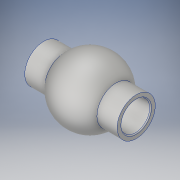
# Autodesk Inventor part: Bola_de_libertad_menor
Saved by Autodesk Inventor 2019 (Build 230136000, 136)
## iProperties
Created: 2019-09-21
Part Number: Bola_de_libertad_menor
Material: Aluminio 6061
Document SubType Name: Modeling
Designer: axelj
Density: 2.7 g/cm^3
Appearance: Aluminio - Plano
Author: axelj
Autodesk Inventor part; units mm, degrees
ref_plane "XZ Plane" through (0, 0, 0) normal (0, 1, 0) x (-1, 0, 0)
ref_plane "XY Plane" through (0, 0, 0) normal (0, 0, 1) x (1, 0, 0)
sketch "Boceto1" plane through (0, 0, 0) normal (1, 0, 0) x (0, 1, 0)
  arc A0 (-2.79, 0) -> (2.79, 0) centre (0, 0) ccw
  line L0 (-2.79, 0) -> (2.79, 0)
  dimension "d0" = 5.58
  constraints: 2 end point, 2 point on circle, 1 centre point, 1 coincident, 1 horizontal
  measures "d0" diameter of A0
revolve "Revolución1" add sketch "Boceto1" angle 360 about axis through (0, -2.79, 0) along (0, 1, 0)
ref_plane "Plano de trabajo1" through (2.8, 0, 0) normal (1, 0, 0) x (0, 1, 0)
sketch "Boceto2" plane through (2.8, 0, 0) normal (1, 0, 0) x (0, 1, 0)
  circle A0 centre (0, 0) radius 1.65
  dimension "d3" = 3.3
  constraints: 1 centre point, 1 coincident
  measures "d3" diameter of A0
extrude "Extrusión1" add sketch "Boceto2" along normal blind 1.2 and the other way blind 6.8
sketch "Boceto3" plane through (4, 0, 0) normal (1, 0, 0) x (0, 0, -1)
  circle A0 centre (0, 0) radius 1.65
  circle A1 centre (0, 0) radius 1.25
  dimension "d8" = 2.5
  constraints: 2 centre point, 2 coincident
  measures "d8" diameter of A1
extrude "Extrusión2" cut sketch "Boceto3" against normal blind 13.6 contours A1
fillet "Empalme1" radius 0.08 2 edges at (4, 0, 1.25) (-4, 0, 1.25)
